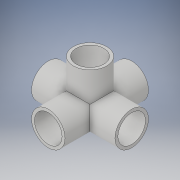
# Autodesk Inventor part: 5-way 1 Inch
Saved by Autodesk Inventor 2018 (Build 220112000, 112)
## iProperties
Created: 2018-01-22
Part Number: 5-way 1 Inch
Material: Generic
Document SubType Name: Modeling
Designer: owner
Density: 1 g/cm^3
Appearance: Default
Author: owner
Autodesk Inventor part; units mm, degrees
ref_plane "YZ Plane" through (0, 0, 0) normal (1, 0, 0) x (0, 1, 0)
sketch "Sketch1" plane through (0, 0, 0) normal (0, 0, 1) x (1, 0, 0)
  circle A0 centre (0, 0) radius 20.3835
  dimension "d0" = 40.767
  constraints: 1 centre point, 1 coincident
  measures "d0" diameter of A0
extrude "Extrusion1" add sketch "Sketch1" against normal blind 101.6
sketch "Sketch2" plane through (0, 0, 0) normal (0, 0, 1) x (1, 0, 0)
  line L0 (0, 0) -> (0, 19.704)
  constraints: 2 end point, 1 vertical
sketch "Sketch3" plane through (0, 0, -101.6) normal (0, 0, -1) x (-1, 0, 0)
  line L0 (0, 0) -> (0, 20.098)
  constraints: 2 end point, 1 vertical
sketch "Sketch11" plane through (0, 0, 0) normal (0, 0, 1) x (1, 0, 0)
  circle A0 centre (0, 0) radius 20.3835 projected
  line L0 (0, 20.3835) -> (23.5166, 20.3835)
  constraints: 2 end point, 2 horizontal, 1 vertical alignment, 1 other
sketch "Sketch12" plane through (0, 0, -101.6) normal (0, 0, -1) x (-1, 0, 0)
  line L0 (0, 20.3509) -> (-24.2704, 20.3509)
  point P0 (0, 0)
  constraints: 2 end point, 1 horizontal
ref_plane "Work Plane1" through (0, 0, 0) normal (-1, 0, 0) x (0, 1, 0)
ref_plane "Work Plane2" through (0, 20.3835, 0) normal (0, 1, -0.0003) x (1, 0, 0)
sketch "Sketch4" plane through (0, 0, 0) normal (-1, 0, 0) x (0, 1, 0)
  circle A0 centre (0, 50.8) radius 20.3835
  point P0 (0, 0)
  constraints: 1 centre point
extrude "Extrusion2" add sketch "Sketch4" along normal mid plane 101.6
sketch "Sketch13" plane through (0, 20.3835, 0) normal (0, 1, -0.0003) x (1, 0, 0)
  ellipse E0 centre (0, 50.8065) end of major axis (20.3835, 30.423) minor radius 0.0046 (0, 50.8131) -> (0, 50.8) ccw projected
  circle A0 centre (0, 50.8) radius 20.3835
  point P0 (0, 0.0065)
  dimension "d23" = 40.767
  constraints: 1 centre point, 1 other
  measures "d23" diameter of A0
extrude "Extrusion9" add sketch "Sketch13" along normal blind 30.4165 and the other way blind 20.3835
sketch "Sketch5" plane through (0, 0, 0) normal (0, 0, 1) x (1, 0, 0)
  circle A0 centre (0, 0) radius 16.7767
  dimension "d5" = 33.5534
  constraints: 1 centre point, 1 coincident
  measures "d5" diameter of A0
sketch "Sketch6" plane through (50.8, 0, -50.8) normal (1, 0, 0) x (0, 0, -1)
  circle A0 centre (0, 0) radius 16.7767
  point P0 (-50.8, 0)
  dimension "d6" = 33.5534
  constraints: 1 centre point
  measures "d6" diameter of A0
sketch "Sketch7" plane through (0, 0, -101.6) normal (0, 0, -1) x (-1, 0, 0)
  circle A0 centre (0, 0) radius 20.3835 projected
  circle A1 centre (0, 0) radius 16.7767
  dimension "d7" = 33.5534
  constraints: 1 centre point, 1 coincident
  measures "d7" diameter of A1
sketch "Sketch8" plane through (-50.8, 0, -50.8) normal (-1, 0, 0) x (0, 0, 1)
  circle A0 centre (0, 0) radius 16.7767
  point P0 (50.8, 0)
  dimension "d8" = 33.5534
  constraints: 1 centre point
  measures "d8" diameter of A0
extrude "Extrusion3" cut sketch "Sketch5" against normal blind 31.75
extrude "Extrusion4" cut sketch "Sketch6" against normal blind 31.75
extrude "Extrusion5" cut sketch "Sketch7" against normal blind 31.75 contours A1
extrude "Extrusion6" cut sketch "Sketch8" against normal blind 31.75
sketch "Sketch9" plane through (0, 0, 0) normal (0, 0, 1) x (1, 0, 0)
  circle A0 centre (0, 0) radius 12.7
  dimension "d17" = 25.4
  constraints: 1 centre point, 1 coincident
  measures "d17" diameter of A0
sketch "Sketch10" plane through (50.8, 0, -50.8) normal (1, 0, 0) x (0, 0, -1)
  circle A0 centre (0, 0) radius 12.7
  point P0 (-50.8, 0)
  dimension "d18" = 25.4
  constraints: 1 centre point
  measures "d18" diameter of A0
extrude "Extrusion7" cut sketch "Sketch10" against normal blind 101.6
extrude "Extrusion8" cut sketch "Sketch9" against normal blind 101.6
sketch "Sketch14" plane through (0, 50.7837, -50.8097) normal (0, 1, -0.0003) x (1, 0, 0)
  ellipse E0 centre (0, 0.0065) end of major axis (20.3835, -20.377) minor radius 0.0046 (0, 0.0131) -> (-14.4124, 14.4143) ccw projected
  circle A0 centre (0, 0.0131) radius 16.7767
  point P0 (0, -50.7935)
  dimension "d28" = 33.5534
  constraints: 1 centre point, 1 other
  measures "d28" diameter of A0
extrude "Extrusion10" cut sketch "Sketch14" against normal blind 31.75
sketch "Sketch15" plane through (0, 50.7837, -50.8097) normal (0, 1, -0.0003) x (1, 0, 0)
  ellipse E0 centre (0, 0.0065) end of major axis (-20.3835, -20.377) minor radius 0.0046 (14.4124, 14.4143) -> (0, 0.0131) ccw projected
  circle A0 centre (0, 0.0131) radius 12.7
  point P0 (0, -50.7935)
  dimension "d31" = 25.4
  constraints: 1 centre point, 1 other
  measures "d31" diameter of A0
extrude "Extrusion11" cut sketch "Sketch15" against normal blind 50.8
body "Solid1"
